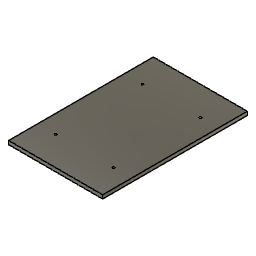
base130_200 v1 (Autodesk Fusion 360 design; units mm, degrees)
Autodesk Fusion 360 part; units mm, degrees
sketch "Sketch1" plane through (0, 0, 0) normal (0, 0, 1) x (1, 0, 0)
  line L0 (0, 0) -> (130, 0)
  line L1 (130, 0) -> (130, 200)
  line L2 (130, 200) -> (0, 200)
  line L3 (0, 200) -> (0, 0)
  circle A0 centre (25, 160) radius 1.5
  circle A1 centre (105, 160) radius 1.5
  circle A2 centre (25, 40) radius 1.5
  circle A3 centre (105, 40) radius 1.5
  dimension "d1" = 130
  dimension "d2" = 200
  dimension "d11" = 3
  dimension "d12" = 3
  dimension "d13" = 3
  dimension "d14" = 3
  constraint horizontal L0
  constraint vertical L1
  constraint horizontal L2
  constraint vertical L3
  constraint coincident L0.start L3.end
  measures "d1" distance of L0.start L0.end
  measures "d2" distance of L0.start L2.end
  measures "d11" diameter of A0
  measures "d12" diameter of A1
  measures "d13" diameter of A2
  measures "d14" diameter of A3
extrude "Extrude1" add sketch "Sketch1" along normal blind 5
